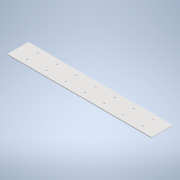
# Autodesk Inventor part: Samle_plade
Saved by Autodesk Inventor 2022 (Build 260153000, 153)
## iProperties
Created: 2022-05-04
Part Number: Samle_plade
Material: Generic
Document SubType Name: Sheet Metal
Designer: Patrick
Density: 1 g/cm^3
Sheet Metal Rule: Default_mm
Appearance: Default
Author: Patrick
Autodesk Inventor part; units mm, degrees
ref_plane "YZ Plane" through (0, 0, 0) normal (1, 0, 0) x (0, 1, 0)
ref_plane "XZ Plane" through (0, 0, 0) normal (0, 1, 0) x (-1, 0, 0)
ref_plane "XY Plane" through (0, 0, 0) normal (0, 0, 1) x (1, 0, 0)
sketch "Sketch1" plane through (0, 0, 0) normal (0, 1, 0) x (-1, 0, 0)
  line L0 (0, 0) -> (300, 0)
  line L1 (300, 0) -> (300, -44)
  line L2 (300, -44) -> (0, -44)
  line L3 (0, -44) -> (0, 0)
  circle A0 centre (270, -11) radius 1.675
  circle A1 centre (270, -33) radius 1.675
  circle A2 centre (230, -11) radius 1.675
  circle A3 centre (230, -33) radius 1.675
  circle A4 centre (190, -11) radius 1.675
  circle A5 centre (190, -33) radius 1.675
  circle A6 centre (150, -11) radius 1.675
  circle A7 centre (150, -33) radius 1.675
  circle A8 centre (110, -11) radius 1.675
  circle A9 centre (110, -33) radius 1.675
  circle A10 centre (70, -11) radius 1.675
  circle A11 centre (70, -33) radius 1.675
  circle A12 centre (30, -11) radius 1.675
  circle A13 centre (30, -33) radius 1.675
  dimension "d0" = 44
  dimension "d1" = 300
  dimension "d2" = 3.35
  dimension "d3" = 11
  dimension "d4" = 3.35
  dimension "d5" = 30
  dimension "d6" = 30
  dimension "d7" = 11
  dimension "d10" = 40
  measures "d0" distance of L2.end L0.start
  measures "d1" distance of L1.end L2.end
  measures "d2" diameter of A0
  measures "d3" distance from line of L0 A0.centre
  measures "d4" diameter of A1
  measures "d5" distance from line of L1 A0.centre
  measures "d6" distance from line of L1 A1.centre
  measures "d7" distance from line of L2 A1.centre
  measures "d10" distance of A0.centre A2.centre
extrude "Plate1" add sketch "Sketch1" along normal blind 1.5
equation "\"d4\" = d2"
equation "\"d15\" = Thickness"
equation "\"BendRadius\" = Thickness"
equation "\"BendReliefWidth\" = Thickness"
equation "\"BendReliefDepth\" = 0.5 * Thickness"
equation "\"CornerReliefSize\" = 4 * Thickness"
equation "\"MinimumRemnant\" = 2 * Thickness"
equation "\"TransitionRadius\" = BendRadius"
equation "\"JacobiRadiusSize\" = BendRadius"
equation "\"GapSize\" = Thickness"
equation "\"Thickness\" = 1.5"
body "Solid1"
